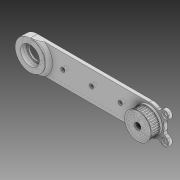
# Autodesk Inventor part: Scara1_top
Saved by Autodesk Inventor 2020 (Build 240168000, 168)
## iProperties
Created: 2020-07-24
Part Number: Scara1_top
Material: Generic
Document SubType Name: Modeling
Designer: DDeGo
Density: 1 g/cm^3
Appearance: Default
Author: DDeGo
Autodesk Inventor part; units mm, degrees
ref_plane "YZ Plane" through (0, 0, 0) normal (1, 0, 0) x (0, 1, 0)
ref_plane "XZ Plane" through (0, 0, 0) normal (0, 1, 0) x (-1, 0, 0)
ref_plane "XY Plane" through (0, 0, 0) normal (0, 0, 1) x (1, 0, 0)
sketch "Sketch1" plane through (0, 0, 0) normal (0, 0, 1) x (1, 0, 0)
  line L0 (-50.15, 0) -> (50.15, 0) construction
  line L1 (-50.15, -13) -> (50.15, -13)
  line L2 (50.15, 13) -> (-50.15, 13)
  arc A0 (-50.15, 13) -> (-50.15, -13) centre (-50.15, 0) ccw
  arc A1 (50.15, -13) -> (50.15, 13) centre (50.15, 0) ccw
  circle A2 centre (-50.15, 0) radius 2.75
  circle A3 centre (50.15, 0) radius 2.75
  circle A4 centre (0, 0) radius 1.75
  circle A5 centre (-25, 0) radius 1.75
  circle A6 centre (25, 0) radius 1.75
  dimension "d0" = 13
  dimension "d1" = 100.3
  dimension "d4" = 5.5
  dimension "d18" = 3.5
  dimension "d19" = 25
  dimension "d20" = 25
  constraints: 8 end point, 7 centre point, 4 point on circle, 4 tangent, 3 coincident, 3 equal radius, 2 point on line, 1 horizontal, 1 midpoint, 1 parallel
  measures "d0" radius of A1
  measures "d1" distance of L0.start L0.end
  measures "d4" diameter of A3
  measures "d18" diameter of A5
  measures "d19" distance of A4.centre A5.centre
  measures "d20" distance of A6.centre A4.centre
extrude "Extrusion1" add sketch "Sketch1" along normal blind 3
sketch "Sketch2" plane through (0, 0, 3) normal (0, 0, 1) x (1, 0, 0)
  circle A0 centre (50.15, 0) radius 2.75 projected
  circle A1 centre (50.15, 0) radius 8.15 construction
  circle A2 centre (50.15, 0) radius 11.5
  arc A3 (50.15, -13) -> (50.15, 13) centre (50.15, 0) ccw projected
  point P0 (0, 0)
  dimension "d6" = 16.3
  dimension "d32" = 23
  constraints: 2 centre point, 2 coincident, 1 concentric
  measures "d6" diameter of A1
  measures "d32" diameter of A2
extrude "Extrusion2" add sketch "Sketch2" along normal blind 10 contours A0 | A2
sketch "Sketch5" plane through (0, 0, 3) normal (0, 0, 1) x (1, 0, 0)
  circle A0 centre (-50.15, 0) radius 2.75 projected
  arc A1 (-50.15, 13) -> (-50.15, -13) centre (-50.15, 0) ccw projected
  circle A2 centre (-50.15, 0) radius 13
  circle A3 centre (-50.15, 0) radius 8.15
  point P0 (0, 0)
  point P1 (-50.15, -13)
  dimension "d21" = 16.3
  constraints: 2 coincident, 1 centre point, 3 other
  measures "d21" diameter of A3
extrude "Extrusion5" add sketch "Sketch5" along normal blind 3.5 contours A2 A1
sketch "Sketch6" plane through (-50.15, 0, 6.5) normal (0, 0, 1) x (1, 0, 0)
  circle A0 centre (0, 0) radius 8.15 projected
  point P0 (50.15, 0)
extrude "Extrusion6" cut sketch "Sketch6" against normal blind 5
sketch "Sketch7" plane through (-50.15, 0, 1.5) normal (0, 0, 1) x (1, 0, 0)
  circle A0 centre (0, 0) radius 2.75 projected
  circle A1 centre (0, 0) radius 8.15 projected
  circle A2 centre (0, 0) radius 6.65
  point P0 (50.15, 0)
  dimension "d26" = 1.5
  constraints: 1 centre point
  measures "d26" radial gap between concentric circles of A1 A2
extrude "Extrusion7" cut sketch "Sketch7" against normal through all contours A2
chamfer "Chamfer2" distance 3 angle 45 1 edges at (-37.15, 0, 3)
ref_plane "Work Plane1" through (50.15, 0, 12) normal (0, 0, 1) x (1, 0, 0)
sketch "Sketch8" plane through (50.15, 0, 12) normal (0, 0, 1) x (1, 0, 0)
  line L0 (0, 0) -> (0, 11.5) construction
  line L1 (0, 0) -> (1.9924, 11.3261) construction
  arc A0 (1.9924, 11.3261) -> (0, 11.5) centre (0, 0) ccw construction
  circle A1 centre (0, 0) radius 11.5 construction
  circle A2 centre (0, 10.9) radius 0.6
  circle A3 centre (0, 0) radius 10.9
  circle A4 centre (-1.8928, 10.7344) radius 0.6
  circle A5 centre (-3.728, 10.2426) radius 0.6
  circle A6 centre (-5.45, 9.4397) radius 0.6
  circle A7 centre (-7.0064, 8.3499) radius 0.6
  circle A8 centre (-8.3499, 7.0064) radius 0.6
  circle A9 centre (-9.4397, 5.45) radius 0.6
  circle A10 centre (-10.2426, 3.728) radius 0.6
  circle A11 centre (-10.7344, 1.8928) radius 0.6
  circle A12 centre (-10.9, 0) radius 0.6
  circle A13 centre (-10.7344, -1.8928) radius 0.6
  circle A14 centre (-10.2426, -3.728) radius 0.6
  circle A15 centre (-9.4397, -5.45) radius 0.6
  circle A16 centre (-8.3499, -7.0064) radius 0.6
  circle A17 centre (-7.0064, -8.3499) radius 0.6
  circle A18 centre (-5.45, -9.4397) radius 0.6
  circle A19 centre (-3.728, -10.2426) radius 0.6
  circle A20 centre (-1.8928, -10.7344) radius 0.6
  circle A21 centre (0, -10.9) radius 0.6
  circle A22 centre (1.8928, -10.7344) radius 0.6
  circle A23 centre (3.728, -10.2426) radius 0.6
  circle A24 centre (5.45, -9.4397) radius 0.6
  circle A25 centre (7.0064, -8.3499) radius 0.6
  circle A26 centre (8.3499, -7.0064) radius 0.6
  circle A27 centre (9.4397, -5.45) radius 0.6
  circle A28 centre (10.2426, -3.728) radius 0.6
  circle A29 centre (10.7344, -1.8928) radius 0.6
  circle A30 centre (10.9, 0) radius 0.6
  circle A31 centre (10.7344, 1.8928) radius 0.6
  circle A32 centre (10.2426, 3.728) radius 0.6
  circle A33 centre (9.4397, 5.45) radius 0.6
  circle A34 centre (8.3499, 7.0064) radius 0.6
  circle A35 centre (7.0064, 8.3499) radius 0.6
  circle A36 centre (5.45, 9.4397) radius 0.6
  circle A37 centre (3.728, 10.2426) radius 0.6
  circle A38 centre (1.8928, 10.7344) radius 0.6
  circle A39 centre (0, 0) radius 14.5061
  point P0 (-50.15, 0)
  point P1 (1.2992, 10.8223)
  point P2 (2.4806, 10.614)
  point P3 (3.1588, 10.4323)
  point P4 (4.286, 10.022)
  point P5 (4.9223, 9.7253)
  point P6 (5.9612, 9.1255)
  point P7 (6.5363, 8.7228)
  point P8 (7.4552, 7.9517)
  point P9 (7.9517, 7.4552)
  point P10 (8.7228, 6.5363)
  point P11 (9.1255, 5.9612)
  point P12 (9.7253, 4.9223)
  point P13 (10.022, 4.286)
  point P14 (10.4323, 3.1588)
  point P15 (10.614, 2.4806)
  point P16 (10.8223, 1.2992)
  point P17 (10.8835, 0.5998)
  point P18 (10.8835, -0.5998)
  point P19 (10.8223, -1.2992)
  point P20 (10.614, -2.4806)
  point P21 (10.4323, -3.1588)
  point P22 (10.022, -4.286)
  point P23 (9.7253, -4.9223)
  point P24 (9.1255, -5.9612)
  point P25 (8.7228, -6.5363)
  point P26 (7.9517, -7.4552)
  point P27 (7.4552, -7.9517)
  point P28 (6.5363, -8.7228)
  point P29 (5.9612, -9.1255)
  point P30 (4.9223, -9.7253)
  point P31 (4.286, -10.022)
  point P32 (3.1588, -10.4323)
  point P33 (2.4806, -10.614)
  point P34 (1.2992, -10.8223)
  point P35 (0.5998, -10.8835)
  point P36 (-0.5998, -10.8835)
  point P37 (-1.2992, -10.8223)
  point P38 (-2.4806, -10.614)
  point P39 (-3.1588, -10.4323)
  point P40 (-4.286, -10.022)
  point P41 (-4.9223, -9.7253)
  point P42 (-5.9612, -9.1255)
  point P43 (-6.5363, -8.7228)
  point P44 (-7.4552, -7.9517)
  point P45 (-7.9517, -7.4552)
  point P46 (-8.7228, -6.5363)
  point P47 (-9.1255, -5.9612)
  point P48 (-9.7253, -4.9223)
  point P49 (-10.022, -4.286)
  point P50 (-10.4323, -3.1588)
  point P51 (-10.614, -2.4806)
  point P52 (-10.8223, -1.2992)
  point P53 (-10.8835, -0.5998)
  point P54 (-10.8835, 0.5998)
  point P55 (-10.8223, 1.2992)
  point P56 (-10.614, 2.4806)
  point P57 (-10.4323, 3.1588)
  point P58 (-10.022, 4.286)
  point P59 (-9.7253, 4.9223)
  point P60 (-9.1255, 5.9612)
  point P61 (-8.7228, 6.5363)
  point P62 (-7.9517, 7.4552)
  point P63 (-7.4552, 7.9517)
  point P64 (-6.5363, 8.7228)
  point P65 (-5.9612, 9.1255)
  point P66 (-4.9223, 9.7253)
  point P67 (-4.286, 10.022)
  point P68 (-3.1588, 10.4323)
  point P69 (-2.4806, 10.614)
  point P70 (-1.2992, 10.8223)
  point P71 (-0.5998, 10.8835)
  point P72 (0.5998, 10.8835)
  dimension "d34" = 2
  dimension "d35" = 9.977
  dimension "d36" = 1.2
  dimension "d37" = 0.6
  dimension "d40" = 360
  constraints: 38 centre point, 4 end point, 4 point on circle, 3 coincident, 1 concentric, 1 point on line, 1 vertical, 76 other
  measures "d34" distance of L0.end L1.end
  measures "d35" angle of L1 L0
  measures "d36" diameter of A2
  measures "d37" distance of L0.end A2.centre
extrude "Extrusion8" cut sketch "Sketch8" against normal blind 7 contours A2 A3 | A3 A2 | A4 A3 | A3 A4 | A38 A3 | A3 A38 | A5 A3 | A3 A5 | A37 A3 | A3 A37 | A6 A3 | A3 A6 | A36 A3 | A3 A36 | A7 A3 | A3 A7 | A35 A3 | A3 A35 | A8 A3 | A3 A8 | A34 A3 | A3 A34 | A9 A3 | A3 A9 | A33 A3 | A3 A33 | A10 A3 | A3 A10 | A32 A3 | A3 A32 | A11 A3 | A3 A11 | A31 A3 | A3 A31 | A12 A3 | A3 A12 | A30 A3 | A3 A30 | A13 A3 | A3 A13 | A29 A3 | A3 A29 | A14 A3 | A3 A14 | A28 A3 | A3 A28 | A15 A3 | A3 A15 | A27 A3 | A3 A27 | A16 A3 | A3 A16 | A26 A3 | A3 A26 | A17 A3 | A3 A17 | A25 A3 | A3 A25 | A18 A3 | A3 A18 | A24 A3 | A3 A24 | A19 A3 | A3 A19 | A23 A3 | A3 A23 | A20 A3 | A3 A20 | A22 A3 | A3 A22 | A21 A3 | A3 A21 | A39
chamfer "Chamfer3" distance 0.6 angle 45 1 edges at (38.65, 0, 12)
sketch "Sketch11" plane through (0, 0, 0) normal (0, 1, 0) x (-1, 0, 0)
  line L0 (-52.9, 0) -> (-47.4, 0) projected
  line L1 (-50.15, 0) -> (-50.15, 13)
  line L2 (-50.15, 13) -> (-52.9, 13)
  line L3 (-38.65, 13) -> (-61.65, 13) projected
  line L4 (-52.85, 4.112) -> (-52.9, 0) construction
  line L5 (-50.15, 0) -> (-50.15, 3) projected
  line L6 (-52.9, 0) -> (-52.9, 13)
  line L7 (-50.15, 0) -> (-52.9, 0)
  point P0 (0, 0)
  constraints: 10 end point, 2 midpoint, 2 perpendicular, 1 vertical
revolve "Revolution1" cut sketch "Sketch11" angle 360 about axis through (50.15, 0, 0) along (0, 0, 1)
sketch "Sketch12" plane through (0, 0, 3) normal (0, 0, 1) x (1, 0, 0)
  arc A0 (50.15, -13) -> (50.15, 13) centre (50.15, 0) ccw projected
  line L0 (63.15, 0) -> (63.5874, 0) construction
  line L1 (63.5874, 0) -> (63.5874, 10) construction
  circle A1 centre (63.5874, 10) radius 1.6
  arc A2 (65.8262, 6.9916) -> (61.3485, 13.0084) centre (63.5874, 10) ccw
  line L2 (65.8262, 6.9916) -> (62.3745, 4.4229)
  line L3 (61.3485, 13.0084) -> (57.8969, 10.4396)
  line L4 (62.3745, 4.4229) -> (57.8969, 10.4396)
  line L5 (63.15, 0) -> (70.6464, 0) construction
  circle A3 centre (63.5874, -10) radius 1.6
  arc A4 (61.3485, -13.0084) -> (65.8262, -6.9916) centre (63.5874, -10) ccw
  line L6 (65.8262, -6.9916) -> (62.3745, -4.4229)
  line L7 (61.3485, -13.0084) -> (57.8969, -10.4396)
  line L8 (62.3745, -4.4229) -> (57.8969, -10.4396)
  point P0 (0, 0)
  point P1 (57.8969, -10.4396)
  dimension "d61" = 3.2
  dimension "d62" = 7.5
  dimension "d64" = 10
  constraints: 18 end point, 7 point on circle, 7 symmetric about line, 4 centre point, 4 coincident, 3 tangent, 2 horizontal, 2 perpendicular, 1 parallel, 2 other
  measures "d61" diameter of A1
  measures "d62" diameter of A2
  measures "d64" distance of L0.end L1.end
extrude "Extrusion10" add sketch "Sketch12" against normal up to surface (3 mm away) contours A0 L6 A4 L7 | A0 L3 A2 L2
fillet "Fillet1" radius 2 4 edges at (57.8969, -10.4396, 1.5) (62.3745, -4.4229, 1.5) (62.3745, 4.4229, 1.5) (57.8969, 10.4396, 1.5)
sketch "Sketch13" plane through (0, 0, 3) normal (0, 0, 1) x (1, 0, 0)
  circle A0 centre (63.5874, 10) radius 1.6 projected
  circle A1 centre (63.5874, 10) radius 3
  circle A2 centre (63.5874, -10) radius 1.6 projected
  circle A3 centre (63.5874, -10) radius 3
  point P0 (0, 0)
  dimension "d68" = 6
  constraints: 2 centre point, 2 coincident, 1 equal radius
  measures "d68" diameter of A1
extrude "Extrusion11" cut sketch "Sketch13" against normal blind 1.5
sketch "Sketch16" plane through (0, 0, 0) normal (0, 0, -1) x (-1, 0, 0)
  circle A0 centre (-50.15, 0) radius 2.75 projected
  line L0 (-54.8265, 0) -> (-52.4883, 4.05)
  line L1 (-52.4883, 4.05) -> (-47.8117, 4.05)
  line L2 (-47.8117, 4.05) -> (-45.4735, 0)
  line L3 (-45.4735, 0) -> (-47.8117, -4.05)
  line L4 (-47.8117, -4.05) -> (-52.4883, -4.05)
  line L5 (-52.4883, -4.05) -> (-54.8265, 0)
  point P0 (0, 0)
  dimension "d91" = 8.1
  constraints: 12 end point, 1 coincident, 1 horizontal, 13 other
  measures "d91" distance between parallel lines of L1 L4
extrude "Extrusion14" cut sketch "Sketch16" against normal blind 9
equation "\"d19\" = d20"
body "Solid1"
